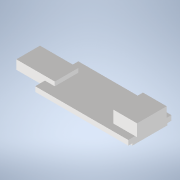
# Autodesk Inventor part: hdmi grabber
Saved by Autodesk Inventor 2022 (Build 260153000, 153)
## iProperties
Created: 2021-11-04
Part Number: hdmi grabber
Material: Generisch
Document SubType Name: Modeling
Designer: lukas
Density: 1 g/cm^3
Appearance: Vorgabe
Author: lukas
Autodesk Inventor part; units mm, degrees
ref_plane "YZ Plane" through (0, 0, 0) normal (1, 0, 0) x (0, 1, 0)
ref_plane "XZ Plane" through (0, 0, 0) normal (0, 1, 0) x (-1, 0, 0)
ref_plane "XY Plane" through (0, 0, 0) normal (0, 0, 1) x (1, 0, 0)
sketch "Skizze2" plane through (0, 0, 0) normal (0, 1, 0) x (-1, 0, 0)
  line L0 (0, 0) -> (47.2, 0)
  line L1 (47.2, 0) -> (47.2, 21.85)
  line L2 (47.2, 21.85) -> (0, 21.85)
  line L3 (0, 21.85) -> (0, 0)
  dimension "d5" = 47.2
  dimension "d6" = 21.85
  constraints: 8 end point, 2 parallel, 1 horizontal, 1 perpendicular
  measures "d5" distance of L2.end L1.end
  measures "d6" distance of L1.end L0.end
extrude "Extrusion2" add sketch "Skizze2" along normal blind 2.5
sketch "Skizze3" plane through (0, 0, 21.85) normal (1, 0, 0) x (0, 0, -1)
  line L0 (3.425, 8.6) -> (18.425, 8.6)
  line L1 (18.425, 8.6) -> (18.425, 2.5)
  line L2 (18.425, 2.5) -> (3.425, 2.5)
  line L3 (3.425, 2.5) -> (3.425, 8.6)
  line L4 (0, 2.5) -> (21.85, 2.5) projected
  point P0 (21.85, 0)
  point P1 (10.925, 2.5)
  point P2 (10.925, 2.5)
  point P3 (10.925, 2.5)
  dimension "d9" = 15
  dimension "d10" = 6.1
  constraints: 8 end point, 3 midpoint, 2 parallel, 1 coincident, 1 horizontal, 1 horizontal alignment, 1 perpendicular
  measures "d9" distance of L0.start L0.end
  measures "d10" distance of L0.end L1.end
extrude "Extrusion3" add sketch "Skizze3" along normal blind 1 and the other way blind 11
sketch "Skizze4" plane through (-47.2, 0, 0) normal (-1, 0, 0) x (0, 0, 1)
  line L0 (4.925, 4.6) -> (16.925, 4.6)
  line L1 (16.925, 4.6) -> (16.925, 0)
  line L2 (16.925, 0) -> (4.925, 0)
  line L3 (4.925, 0) -> (4.925, 4.6)
  line L4 (0, 0) -> (21.85, 0) projected
  point P0 (10.925, 0)
  point P1 (10.925, 0)
  point P2 (10.925, 0)
  dimension "d15" = 12
  dimension "d16" = 4.6
  constraints: 8 end point, 3 midpoint, 2 coincident, 2 parallel, 1 horizontal, 1 perpendicular
  measures "d15" distance of L1.end L2.end
  measures "d16" distance of L0.end L1.end
extrude "Extrusion4" add sketch "Skizze4" along normal blind 14.5 and the other way blind 5
sketch "Skizze5" plane through (0, 0, 0) normal (0, -1, 0) x (1, 0, 0)
  line L0 (-47.2, 17.425) -> (-41, 17.425)
  line L1 (-41, 17.425) -> (-41, 4.425)
  line L2 (-41, 4.425) -> (-47.2, 4.425)
  line L3 (-47.2, 4.425) -> (-47.2, 17.425)
  line L4 (-47.2, 16.925) -> (-61.7, 16.925) projected
  line L5 (-47.2, 4.925) -> (-61.7, 4.925) projected
  line L6 (0, 21.85) -> (0, 0) projected
  line L7 (-11.5, 19.85) -> (0, 19.85)
  line L8 (0, 19.85) -> (0, 2)
  line L9 (0, 2) -> (-11.5, 2)
  line L10 (-11.5, 2) -> (-11.5, 19.85)
  line L11 (-47.2, 21.85) -> (0, 21.85) projected
  line L12 (0, 0) -> (-47.2, 0) projected
  point P0 (0, 19.85)
  dimension "d21" = 6.2
  dimension "d22" = 13
  dimension "d23" = 0.5
  dimension "d24" = 0.5
  dimension "d25" = 11.5
  dimension "d26" = 2
  dimension "d27" = 2
  constraints: 16 end point, 4 parallel, 2 horizontal, 2 perpendicular, 1 point on line, 1 vertical alignment
  measures "d21" distance between parallel lines of L3 L1
  measures "d22" distance between parallel lines of L2 L0
  measures "d23" distance between parallel lines of L4 L0
  measures "d24" distance between parallel lines of L5 L2
  measures "d25" distance of L7.start L7.end
  measures "d26" distance between parallel lines of L11 L7
  measures "d27" distance between parallel lines of L12 L9
extrude "Extrusion5" add sketch "Skizze5" along normal blind 1
equation "\"d23\" = d24"
